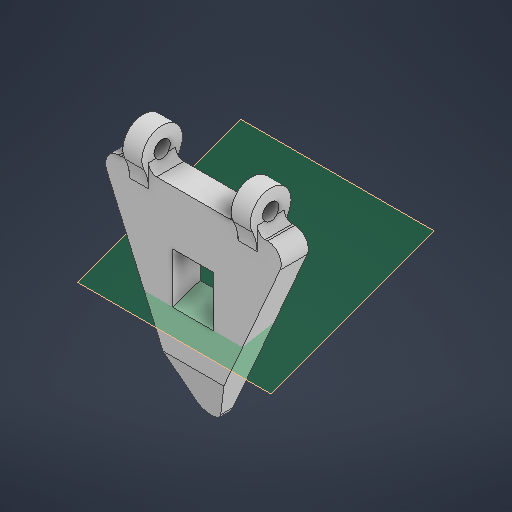
# Autodesk Inventor part: trojúhleník
Saved by Autodesk Inventor 2026 (Build 300175050, 175E)
## iProperties
Created: 2026-02-24
Part Number: trojúhleník
Material: Všeobecné
Document SubType Name: Modeling
Designer: marti
Density: 1 g/cm^3
Appearance: Výchozí
Author: marti
Autodesk Inventor part; units mm, degrees
ref_plane "XZ Plane" through (0, 0, 0) normal (0, 1, 0) x (-1, 0, 0)
ref_plane "XY Plane" through (0, 0, 0) normal (0, 0, 1) x (1, 0, 0)
sketch "Náčrt1" plane through (0, 0, 0) normal (0, 0, 1) x (1, 0, 0)
  line L0 (-35, 35) -> (35, 35)
  line L1 (-35, 35) -> (0, -45)
  line L2 (0, -45) -> (35, 35)
  line L3 (0, 60.6) -> (0, -62.6) projected
  line L4 (-49, 0) -> (49, 0) projected
  line L5 (7.5, 0) -> (-7.5, 0)
  line L6 (-7.5, 0) -> (-7.5, 15)
  line L7 (-7.5, 15) -> (7.5, 15)
  line L8 (7.5, 15) -> (7.5, 0)
  line L9 (7.5, 0) -> (-7.5, 15) construction
  line L10 (-7.5, 0) -> (7.5, 15) construction
  point P0 (0, 0)
  point P1 (0, 7.5)
  dimension "d3" = 70
  dimension "d36" = 80
  dimension "d37" = 35
  dimension "d61" = 15
  dimension "d62" = 15
  dimension "d63" = 20
  constraints: 18 end point, 3 parallel, 2 midpoint, 2 point on line, 1 horizontal, 1 perpendicular, 1 symmetric about line
  measures "d3" distance of L0.start L0.end
  measures "d36" distance from line of L0 L1.end
  measures "d37" distance between parallel lines of L0 L4
  measures "d61" distance of L6.end L7.end
  measures "d62" distance of L5.end L6.end
  measures "d63" distance between parallel lines of L0 L7
extrude "Vysunutí1" add sketch "Náčrt1" along normal mid plane 10 contours L0 L3 L7 L6 L4 L1 | L0 L2 L4 L8 L7 L3 | L4 L3 L1 | L3 L4 L2
fillet "Zaoblení1" radius 5 3 edges at (-35, 35, 0) (35, 35, 0) (0, -45, 0)
ref_plane "Pracovní rovina1" through (20, 0, 0) normal (1, 0, 0) x (0, 1, 0)
ref_plane "Pracovní rovina2" through (-20, 0, 0) normal (1, 0, 0) x (0, 1, 0)
sketch "Náčrt3" plane through (20, 0, 0) normal (1, 0, 0) x (0, 1, 0)
  circle A0 centre (40, 0) radius 7.5
  point P0 (0, 0)
  dimension "d58" = 15
  constraints: 1 centre point, 1 coincident
  measures "d58" diameter of A0
extrude "Vysunutí3" add sketch "Náčrt3" along normal mid plane 7
fillet "Zaoblení2" radius 3 1 edges at (16.5, 35, 0)
mirror "Zrcadlit1" about plane through (0, 0, 0) normal (1, 0, 0) of "Vysunutí3", "Zaoblení2"
ref_plane "Pracovní rovina5" through (0, -19.3577, 5) normal (0, -0.3420201, 0.9396926) x (1, 0, 0)
sketch "Náčrt5" plane through (23.5, 0, 0) normal (1, 0, 0) x (0, 0, -1)
  line L0 (5, 35) -> (-5, 35) projected
  line L1 (-5, 35) -> (-5, 34.4098) projected
  line L2 (5, 34.4098) -> (5, 35) projected
  arc A0 (5, 34.4098) -> (-5, 34.4098) centre (0, 40) ccw projected
  point P0 (0, 0)
hole "Díra1" at (23.5, 40, 0) direction (-1, 0, 0) diameter 6 end through all
sketch "Náčrt8" plane through (0, 0, 0) normal (1, 0, 0) x (0, 1, 0)
  line L0 (-50.0356, 0) -> (58.5059, 0) projected
  line L1 (0, 28.7908) -> (0, -8.2985) projected
  line L2 (27.9959, 5) -> (-34.5296, 5) projected
  arc A0 (38, -2.2361) -> (38, 2.2361) centre (40, 0) ccw projected
  line L3 (40, 0) -> (31.4495, 23.4923)
  line L4 (31.4495, 23.4923) -> (-33.0951, 0)
  line L5 (-33.0951, 0) -> (40, 0)
  point P0 (0, 0)
  point P1 (-19.3577, 5)
  point P2 (0, 5)
  dimension "d47" = 25
  dimension "d48" = 20
  dimension "d49" = 90
  dimension "d50" = 0
  constraints: 6 end point, 1 perpendicular
  measures "d47" distance of L3.start L3.end
  measures "d48" angle of L4 L5
  measures "d49" angle of L4 L3
  measures "d50" distance between parallel lines of L0 L5
sketch "Náčrt9" plane through (0, -19.3577, 5) normal (0, -0.3420201, 0.9396926) x (1, 0, 0)
  line L0 (-61.9016, 55.6047) -> (51.7784, 55.6047)
  line L1 (51.7784, 55.6047) -> (51.7784, -27.5691)
  line L2 (51.7784, -27.5691) -> (-61.9016, -27.5691)
  line L3 (-61.9016, -27.5691) -> (-61.9016, 55.6047)
  point P0 (0, 16.4802)
  constraints: 8 end point, 2 parallel, 1 horizontal, 1 perpendicular
extrude "Vysunutí6" cut sketch "Náčrt9" along normal blind 10
fillet "Zaoblení3" radius 3 2 edges at (23.5, 35, 0) (-23.5, 35, 0)
fillet "Zaoblení4" radius 15 4 edges at (20, 34.4098, -5) (-20, 34.4098, -5) (20, 34.4098, 5) (-20, 34.4098, 5)
ref_plane "Pracovní rovina6" through (7.5, 0, -5) normal (0, -0.9396926, -0.3420201) x (1, 0, 0)
sketch "Náčrt11" plane through (7.5, 0, -5) normal (0, -0.9396926, -0.3420201) x (1, 0, 0)
  line L0 (0, -20.4385) -> (-15, -20.4385)
  line L1 (-15, -20.4385) -> (-15, 29.8354)
  line L2 (-15, 29.8354) -> (0, 29.8354)
  line L3 (0, 29.8354) -> (0, -20.4385)
  line L4 (0, -20.4385) -> (-15, 29.8354) construction
  line L5 (-15, -20.4385) -> (0, 29.8354) construction
  point P0 (-7.5, 4.6985)
  constraints: 12 end point, 2 midpoint, 2 parallel, 1 horizontal, 1 perpendicular
extrude "Vysunutí7" cut sketch "Náčrt11" against normal blind 15
